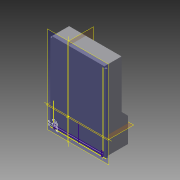
# Autodesk Inventor part: batteri
Saved by Autodesk Inventor 2015 (Build 190159000, 159)
## iProperties
Created: 2015-12-13
Part Number: batteri
Material: Generic
Document SubType Name: Modeling
Designer: abberik
Density: 1 g/cm^3
Appearance: Default
Mass: 35.2422 g
Surface Area: 357.302 cm^2
Volume: 35.2422 cm^3
Author: abberik
Autodesk Inventor part; units mm, degrees
sketch "Sketch1" plane through (0, 0, 0) normal (0, 1, 0) x (-1, 0, 0)
  line L0 (22.3723, -21.9307) -> (-45.6277, -21.9307)
  line L1 (-45.6277, -21.9307) -> (-45.6277, 74.5693)
  line L2 (-45.6277, 74.5693) -> (22.3723, 74.5693)
  line L3 (22.3723, 74.5693) -> (22.3723, -21.9307)
  point P0 (0, 0)
  dimension "d0" = 68
  dimension "d1" = 96.5
  constraints: 8 end point, 2 parallel, 1 horizontal, 1 perpendicular
  measures "d0" distance between parallel lines of L1 L3
  measures "d1" distance between parallel lines of L0 L2
extrude "Extrusion1" add sketch "Sketch1" along normal blind 2
sketch "Sketch3" plane through (0, 2, 0) normal (0, 1, 0) x (1, 0, 0)
  line L0 (-20.3723, 21.9307) -> (43.6277, 21.9307)
  line L1 (43.6277, 21.9307) -> (43.6277, -72.5693)
  line L2 (-20.3723, -72.5693) -> (-20.3723, 21.9307)
  line L3 (45.6277, 21.9307) -> (-22.3723, 21.9307) projected
  line L4 (-22.3723, 21.9307) -> (-22.3723, -74.5693) projected
  line L5 (-22.3723, -74.5693) -> (45.6277, -74.5693) projected
  line L6 (45.6277, -74.5693) -> (45.6277, 21.9307) projected
  line L7 (-20.3723, -72.5693) -> (-20.3723, -74.5693)
  line L8 (-22.3723, -74.5693) -> (45.6277, -74.5693) projected
  line L9 (43.6277, -74.5693) -> (43.6277, -72.5693)
  line L10 (-18.3723, -72.5693) -> (41.6277, -72.5693)
  line L11 (41.6277, -72.5693) -> (41.6277, 21.9307)
  line L12 (41.6277, 21.9307) -> (-18.3723, 21.9307)
  line L13 (-18.3723, 21.9307) -> (-18.3723, -72.5693)
  point P0 (0, 0)
  dimension "d4" = 0
  dimension "d5" = 2
  dimension "d7" = 2
  dimension "d8" = 0
  dimension "d9" = 2
  dimension "d10" = 2
  dimension "d11" = 2
  constraints: 18 end point, 4 perpendicular, 3 parallel, 2 horizontal, 2 point on line
  measures "d4" distance between parallel lines of L3 L0
  measures "d5" distance between parallel lines of L6 L1
  measures "d7" distance between parallel lines of L4 L2
  measures "d8" distance between parallel lines of L0 L12
  measures "d9" distance between parallel lines of L2 L13
  measures "d10" distance between parallel lines of L1 L11
  measures "d11" distance between parallel lines of L5 L10
extrude "Extrusion2" add sketch "Sketch3" along normal blind 25 contours L0 L13 L10 L11 L1 L9 L5 L7 L2
sketch "Sketch4" plane through (0, 27, 0) normal (0, 1, 0) x (1, 0, 0)
  line L0 (41.6277, 21.9307) -> (41.6277, -72.5693) projected
  line L1 (41.6277, -72.5693) -> (-18.3723, -72.5693) projected
  line L2 (-18.3723, -72.5693) -> (-18.3723, 21.9307) projected
  line L3 (-18.3723, 21.9307) -> (-20.3723, 21.9307) projected
  line L4 (-20.3723, 21.9307) -> (-20.3723, -74.5693) projected
  line L5 (-20.3723, -74.5693) -> (43.6277, -74.5693) projected
  line L6 (43.6277, -74.5693) -> (43.6277, 21.9307) projected
  line L7 (43.6277, 21.9307) -> (41.6277, 21.9307) projected
  line L8 (-20.3723, 21.9307) -> (43.6277, 21.9307)
  line L9 (43.6277, 21.9307) -> (43.6277, -74.5693)
  line L10 (43.6277, -74.5693) -> (-20.3723, -74.5693)
  line L11 (-20.3723, -74.5693) -> (-20.3723, 21.9307)
  point P0 (0, 0)
  constraints: 8 end point, 2 parallel, 1 horizontal, 1 perpendicular
extrude "Extrusion3" add sketch "Sketch4" along normal blind 2
sketch "Sketch5" plane through (0, 2, 0) normal (0, 1, 0) x (1, 0, 0)
  line L0 (43.6277, 21.9307) -> (43.6277, -74.5693) projected
  line L1 (43.6277, -74.5693) -> (45.6277, -74.5693) projected
  line L2 (45.6277, -74.5693) -> (45.6277, 21.9307) projected
  line L3 (45.6277, 21.9307) -> (43.6277, 21.9307) projected
  line L4 (-20.3723, -74.5693) -> (-20.3723, 21.9307) projected
  line L5 (-20.3723, 21.9307) -> (-22.3723, 21.9307) projected
  line L6 (-22.3723, 21.9307) -> (-22.3723, -74.5693) projected
  line L7 (-22.3723, -74.5693) -> (-20.3723, -74.5693) projected
  line L8 (-22.3723, -74.5693) -> (-20.3723, -74.5693)
  line L9 (-20.3723, -74.5693) -> (-20.3723, -72.5693)
  line L10 (-20.3723, -72.5693) -> (-22.3723, -72.5693)
  line L11 (-22.3723, -72.5693) -> (-22.3723, -74.5693)
  line L12 (43.6277, -74.5693) -> (43.6277, 21.9307) projected
  line L13 (45.6277, -74.5693) -> (43.6277, -74.5693)
  line L14 (43.6277, -74.5693) -> (43.6277, -72.5693)
  line L15 (43.6277, -72.5693) -> (45.6277, -72.5693)
  line L16 (45.6277, -72.5693) -> (45.6277, -74.5693)
  point P0 (0, 0)
  dimension "d16" = 2
  dimension "d17" = 2
  constraints: 16 end point, 4 parallel, 2 horizontal, 2 perpendicular, 1 point on line
  measures "d16" distance of L10.end L9.end
  measures "d17" distance of L9.end L8.end
extrude "Extrusion4" cut sketch "Sketch5" against normal blind 2 contours L15 L2 L1 L0 | L7 L6 L10 L4
sketch "Sketch6" plane through (-20.3723, 0, 74.5693) normal (-1, 0, 0) x (0, 0, 1)
  line L0 (-96.5, 29) -> (-69.5, 29)
  line L1 (-96.5, 29) -> (0, 29) projected
  line L2 (0, 0) -> (0, 29) projected
  line L3 (0, 19) -> (-59.5, 19)
  line L4 (-69.5, 29) -> (-59.5, 19)
  line L5 (-69.5, 29) -> (-55.3579, 29) construction
  line L6 (-69.5, 29) -> (0, 29)
  line L7 (0, 29) -> (0, 19)
  point P0 (-74.5693, 0)
  dimension "d20" = 27
  dimension "d21" = 10
  dimension "d22" = 45
  constraints: 12 end point, 3 horizontal, 2 point on line, 1 collinear, 1 equal length
  measures "d20" distance of L0.start L0.end
  measures "d21" distance between parallel lines of L1 L3
  measures "d22" angle of L4 L5
extrude "Extrusion5" cut sketch "Sketch6" against normal up to next
sketch "Sketch7" plane through (-20.3723, 2, -21.9307) normal (-1, 0, 0) x (0, 0, 1)
  line L0 (37, 17) -> (27, 27) projected
  line L1 (96.5, 17) -> (37, 17) projected
  line L2 (29.8284, 27) -> (37.8284, 19)
  line L3 (37.8284, 19) -> (96.5, 19)
  line L4 (27, 27) -> (29.8284, 27)
  line L5 (96.5, 17) -> (96.5, 19)
  point P0 (21.9307, -2)
  dimension "d25" = 2
  constraints: 8 end point, 1 horizontal, 1 vertical
  measures "d25" distance between parallel lines of L0 L2
extrude "Extrusion6" add sketch "Sketch7" against normal up to surface (64 mm away)
sketch "Sketch13" plane through (-20.3723, 2, -21.9307) normal (-1, 0, 0) x (0, 0, 1)
  line L0 (6, 2.4048) -> (16, 2.4048)
  line L1 (16, 2.4048) -> (16, 17.4048)
  line L2 (16, 17.4048) -> (6, 17.4048)
  line L3 (6, 17.4048) -> (6, 2.4048)
  line L4 (0, 0) -> (0, 27) projected
  point P0 (21.9307, -2)
  dimension "d46" = 10
  dimension "d47" = 15
  dimension "d50" = 6
  constraints: 8 end point, 2 parallel, 1 horizontal, 1 perpendicular
  measures "d46" distance of L2.end L1.end
  measures "d47" distance of L1.end L0.end
  measures "d50" distance between parallel lines of L4 L3
extrude "Extrusion7" cut sketch "Sketch13" against normal blind 2
sketch "Sketch14" plane through (0, 0, 0) normal (0, -1, 0) x (1, 0, 0)
  line L0 (-18.3723, 7.0693) -> (-18.3723, -21.9307) projected
  line L1 (41.6277, -21.9307) -> (41.6277, 7.0693) projected
  line L2 (-18.3723, -21.9307) -> (-16.3723, -21.9307)
  line L3 (-16.3723, -21.9307) -> (-16.3723, -19.9307)
  line L4 (-16.3723, -19.9307) -> (-18.3723, -19.9307)
  line L5 (-18.3723, -19.9307) -> (-18.3723, -21.9307)
  line L6 (-18.3723, -17.9307) -> (-16.3723, -17.9307)
  line L7 (-16.3723, -17.9307) -> (-16.3723, -15.9307)
  line L8 (-16.3723, -15.9307) -> (-18.3723, -15.9307)
  line L9 (-18.3723, -15.9307) -> (-18.3723, -17.9307)
  line L10 (-22.3723, -21.9307) -> (45.6277, -21.9307) projected
  line L11 (11.6277, -21.9307) -> (11.6277, 0)
  line L12 (39.6277, -21.9307) -> (39.6277, -19.9307)
  line L13 (39.6277, -19.9307) -> (41.6277, -19.9307)
  line L14 (41.6277, -17.9307) -> (39.6277, -17.9307)
  line L15 (39.6277, -17.9307) -> (39.6277, -15.9307)
  line L16 (39.6277, -15.9307) -> (41.6277, -15.9307)
  line L17 (39.6277, -21.9307) -> (41.6277, -21.9307)
  line L18 (41.6277, -19.9307) -> (41.6277, -21.9307)
  line L19 (41.6277, -17.9307) -> (41.6277, -15.9307)
  line L20 (41.6277, -19.9307) -> (41.6277, -17.9307)
  line L21 (39.6277, -17.9307) -> (39.6277, -19.9307)
  line L22 (-16.3723, -19.9307) -> (-16.3723, -17.9307)
  line L23 (-18.3723, -17.9307) -> (-18.3723, -19.9307)
  line L24 (-18.3723, -19.9307) -> (-16.3723, -19.9307)
  line L25 (-16.3723, -19.9307) -> (39.6277, -19.9307)
  line L26 (41.6277, 72.5693) -> (41.6277, -21.9307) projected
  line L27 (39.6277, -17.9307) -> (-16.3723, -17.9307)
  point P0 (0, 0)
  dimension "d51" = 2
  dimension "d52" = 2
  dimension "d53" = 2
  dimension "d54" = 2
  dimension "d55" = 2
  constraints: 48 end point, 7 symmetric about line, 5 parallel, 4 collinear, 4 perpendicular, 3 horizontal, 1 midpoint, 1 point on line, 1 vertical
  measures "d51" distance of L4.end L3.end
  measures "d52" distance of L3.end L2.end
  measures "d53" distance of L8.end L7.end
  measures "d54" distance of L7.end L6.end
  measures "d55" distance between parallel lines of L6 L4
extrude "Extrusion8" add sketch "Sketch14" against normal up to surface (27 mm away) contours L8 L7 L6 L0 | L4 L3 L2 L0 | L15 L16 L1 L14 | L13 L1 L10 L12
extrude "Extrusion10" cut sketch "Sketch14" against normal up to next contours L6 L22 L4 L0 | L27 L11 L25 L22 | L27 L21 L25 L11 | L14 L1 L13 L21
body "Solid1"
